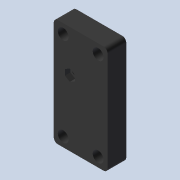
# Autodesk Inventor part: 10_Mountinplate_Mirrors_v1_Combiner
Saved by Autodesk Inventor 2022 (Build 260153000, 153)
## iProperties
Created: 2022-05-18
Part Number: 10_Mountinplate_Mirrors_v1_Combiner
Material: Generisch
Document SubType Name: Modeling
Designer: diederichbenedict
Density: 1 g/cm^3
Appearance: Vorgabe
Author: diederichbenedict
Autodesk Inventor part; units mm, degrees
ref_plane "Arbeitsebene1" through (0.0075, -0.0423, 0) normal (0, 0, 1) x (1, 0, 0)
sketch "Skizze1" plane through (0.0075, -0.0423, 0) normal (0, 0, 1) x (1, 0, 0)
  line L0 (0.635, 25.527) -> (10.16, 25.527) projected
  line L1 (0.635, 25.527) -> (0.635, 0) projected
  line L2 (0.635, 0) -> (10.16, 0) projected
  line L3 (10.16, 0) -> (10.16, 25.527) projected
  line L4 (30.08, -27.3) -> (-3.92, -27.3)
  line L5 (-6.92, -24.3) -> (-6.92, 49.7)
  line L6 (-3.92, 52.7) -> (30.08, 52.7)
  line L7 (33.08, -27.3) -> (-6.92, 52.7) construction
  line L8 (-6.92, -27.3) -> (33.08, 52.7) construction
  arc A0 (30.08, -27.3) -> (33.08, -24.3) centre (30.08, -24.3) ccw
  arc A1 (-6.92, -24.3) -> (-3.92, -27.3) centre (-3.92, -24.3) ccw
  arc A2 (-3.92, 52.7) -> (-6.92, 49.7) centre (-3.92, 49.7) ccw
  arc A3 (33.08, 49.7) -> (30.08, 52.7) centre (30.08, 49.7) ccw
  circle A4 centre (5.08, 12.7) radius 2.3813
  line L9 (33.08, -24.3) -> (33.08, 49.7)
  line L10 (5.08, 12.7) -> (5.08, 21.7)
  line L11 (5.08, 12.7) -> (14.08, 12.7) construction
  circle A5 centre (5.08, 21.7) radius 2.3813
  point P0 (-0.0075, 0.0423)
  point P1 (13.08, 12.7)
  dimension "d1" = 80
  dimension "d2" = 3
  dimension "d7" = 0
  dimension "d8" = 8
  dimension "d41" = 9
  dimension "d42" = 90
  constraints: 16 end point, 8 point on circle, 7 tangent, 6 centre point, 6 point on line, 3 equal radius, 2 horizontal, 2 perpendicular, 2 vertical, 1 midpoint, 1 parallel, 2 other
  measures "d1" distance of L8.start L7.end
  measures "d2" radius of A0
  measures "d7" vertical distance of L10.start point (13.08, 12.7)
  measures "d8" distance of point (13.08, 12.7) L10.start
  measures "d41" distance of L10.start L10.end
  measures "d42" angle of L11 L10
ref_plane "Arbeitsebene2" through (291.5074, -13.3966, 8.6065) normal (0, 0, 1) x (0.898794, -0.4383711, 0)
extrude "Extrusion1" add sketch "Skizze1" along normal blind 12.612 contours L0 L3 L2 L1 | L4 A1 L5 A2 L6 A3 L9 A0 | A4
sketch "Skizze3" plane through (0.0075, -0.0423, 0) normal (0, 0, -1) x (-1, 0, 0)
  arc A0 (-30.08, 52.7) -> (-33.08, 49.7) centre (-30.08, 49.7) ccw projected
  line L0 (-33.08, -24.3) -> (-33.08, 49.7) projected
  arc A1 (-33.08, -24.3) -> (-30.08, -27.3) centre (-30.08, -24.3) ccw projected
  line L1 (3.92, -27.3) -> (-30.08, -27.3) projected
  arc A2 (3.92, -27.3) -> (6.92, -24.3) centre (3.92, -24.3) ccw projected
  line L2 (6.92, 49.7) -> (6.92, -24.3) projected
  arc A3 (6.92, 49.7) -> (3.92, 52.7) centre (3.92, 49.7) ccw projected
  line L3 (-30.08, 52.7) -> (3.92, 52.7) projected
  line L4 (-26.08, 45.7) -> (-0.08, 45.7)
  line L5 (-0.08, 45.7) -> (-0.08, -20.3)
  line L6 (-0.08, -20.3) -> (-26.08, -20.3)
  line L7 (-26.08, -20.3) -> (-26.08, 45.7)
  point P0 (0.0075, 0.0423)
  dimension "d9" = 7
  constraints: 8 end point, 3 other
  measures "d9" distance between parallel lines of L0 L7
hole "Bohrung1" at (26.0875, 45.6577, 0) at (26.0875, -20.3423, 0) at (0.0875, -20.3423, 0) at (0.0875, 45.6577, 0) direction (0, 0, 1) diameter 8 depth 15 tip angle 118
sketch "Skizze4" plane through (-6.9125, -24.3423, 0) normal (-1, 0, 0) x (0, 0, 1)
  circle A0 centre (-6.731, 17.9923) radius 7.366 projected
  circle A1 centre (-6.731, 17.9923) radius 9.366
  circle A2 centre (-6.731, 56.05) radius 7.366
  circle A3 centre (-6.731, 56.05) radius 9.366
  line L0 (-6.731, 17.9923) -> (-6.731, 26.9923)
  line L1 (-6.731, 17.9923) -> (2.269, 17.9923) construction
  circle A4 centre (-6.731, 26.9923) radius 9.366
  point P0 (0, 24.3423)
  dimension "d17" = 2
  dimension "d45" = 9
  dimension "d46" = 90
  constraints: 4 centre point, 4 end point, 1 equal radius, 1 horizontal, 1 perpendicular, 1 vertical, 2 other
  measures "d17" radial gap between concentric circles of A0 A1
  measures "d45" distance of L0.start L0.end
  measures "d46" angle of L1 L0
ref_plane "Arbeitsebene3" through (0, -11.176, -49.276) normal (-1, 0, 0) x (0, 0.0000004, 1)
extrude "Extrusion2" cut sketch "Skizze4" against normal up to surface (6.9125 mm away) contours A4 A0 | A0 A4 A1 | A1 A4 picked at (-6.731, 20.2469) picked at (0.3309, 22.9964)
sketch "Skizze5" plane through (0.0075, -0.0423, 0) normal (0, 0, -1) x (-1, 0, 0)
  line L0 (0.0075, -3.8204) -> (0.0075, 9.2051) projected
  arc A0 (6.92, 49.7) -> (3.92, 52.7) centre (3.92, 49.7) ccw projected
  line L1 (-30.08, 52.7) -> (3.92, 52.7) projected
  arc A1 (-30.08, 52.7) -> (-33.08, 49.7) centre (-30.08, 49.7) ccw projected
  line L2 (-33.08, -24.3) -> (-33.08, 49.7) projected
  arc A2 (-33.08, -24.3) -> (-30.08, -27.3) centre (-30.08, -24.3) ccw projected
  line L3 (3.92, -27.3) -> (-30.08, -27.3) projected
  arc A3 (3.92, -27.3) -> (6.92, -24.3) centre (3.92, -24.3) ccw projected
  line L4 (6.92, 49.7) -> (6.92, 9.2051) projected
  circle A4 centre (-0.08, 45.7) radius 4 projected
  circle A5 centre (-26.08, -20.3) radius 4 projected
  circle A6 centre (-26.08, 45.7) radius 4 projected
  circle A7 centre (-0.08, -20.3) radius 4 projected
  line L5 (-0.6275, 29.1761) -> (-10.1525, 29.1761) projected
  line L6 (-0.6275, -2.2391) -> (-10.1525, -2.2391) projected
  line L7 (-10.1525, -2.2391) -> (-10.1525, 29.1761)
  line L8 (-0.6275, 29.1761) -> (-0.6275, -2.2391)
  line L9 (0.0075, 0.2051) -> (0.0075, -12.8204) projected
  line L10 (-10.3525, 29.3761) -> (-0.4275, 29.3761)
  line L11 (-0.4275, 29.3761) -> (-0.4275, -2.4391)
  line L12 (-0.4275, -2.4391) -> (-10.3525, -2.4391)
  line L13 (-10.3525, -2.4391) -> (-10.3525, 29.3761)
  line L14 (6.92, -3.8204) -> (6.92, -24.3) projected
  line L15 (-12.6873, 36.83) -> (-19.1643, 36.83)
  line L16 (-12.6873, -11.811) -> (-19.1643, -11.811)
  line L17 (-12.6873, 17.399) -> (-12.6873, 4.5974)
  line L18 (-19.7993, 21.1275) -> (-19.7993, 26.543)
  line L19 (-12.6873, -11.811) -> (-19.7993, -11.811)
  line L20 (-19.7993, -11.811) -> (-19.7993, 36.83)
  line L21 (-19.7993, 36.83) -> (-12.6873, 36.83)
  line L22 (-12.6873, 36.83) -> (-12.6873, -11.811)
  line L23 (-19.9993, 37.03) -> (-19.9993, -12.011)
  line L24 (-19.9993, -12.011) -> (-12.4873, -12.011)
  line L25 (-12.4873, -12.011) -> (-12.4873, 37.03)
  line L26 (-12.4873, 37.03) -> (-19.9993, 37.03)
  line L27 (-19.9993, -12.011) -> (-22.9993, -12.011)
  line L28 (-22.9993, -12.011) -> (-22.9993, 37.03)
  line L29 (-22.9993, 37.03) -> (-19.9993, 37.03)
  line L30 (-19.9993, 37.03) -> (-19.9993, -12.011)
  line L31 (0, -0.127) -> (0, 25.4)
  line L32 (0, -0.127) -> (0, 25.4)
  line L33 (-0.4275, -2.4391) -> (0.0075, -2.4391)
  line L34 (0.2725, 0.2051) -> (0.2725, 25.2373)
  line L35 (0.2725, 29.3761) -> (-0.4275, 29.3761)
  line L36 (-0.4275, 29.3761) -> (-0.4275, -2.4391)
  line L37 (0, 6.611) -> (-10.36, 6.611)
  line L38 (-10.36, 6.611) -> (-10.36, 38.411)
  line L39 (-10.36, 38.411) -> (0, 38.411)
  line L40 (0, 38.411) -> (0, 6.611)
  line L41 (6.92, 49.7) -> (6.92, 9.2051) projected
  line L42 (0.0075, 6.98) -> (0.0075, -2.82)
  line L43 (-10.36, 38.411) -> (-12.4873, 38.411)
  line L44 (-12.4873, 39.411) -> (-12.4873, -2.4391)
  line L45 (-10.36, -2.4391) -> (-10.36, 39.411)
  line L46 (-12.4873, 39.411) -> (-12.4873, 7.611)
  line L47 (-12.4873, 6.611) -> (-10.36, 6.611)
  line L48 (-10.36, 7.611) -> (-10.36, 39.411)
  line L49 (-12.4873, 48) -> (-22.9993, 48)
  line L50 (-22.9993, 48) -> (-22.9993, -3)
  line L51 (-22.9993, -3) -> (-12.4873, -3)
  line L52 (-12.4873, -3) -> (-12.4873, 48)
  line L53 (6.92, -3.8204) -> (0.0075, -3.8204) projected
  line L54 (0.0075, 9.2051) -> (6.92, 9.2051) projected
  line L55 (0, 39.411) -> (0, 38.411)
  point P0 (6.92, 0.2051)
  point P1 (6.92, 25.2373)
  point P2 (-19.9993, 37.03)
  point P3 (0, 29.3761)
  point P4 (-10.3525, 6.611)
  point P5 (0, 6.611)
  point P6 (-10.36, 6.611)
  point P7 (-22.9993, -13)
  point P8 (-19.9993, 37.03)
  point P9 (-19.9993, 37.03)
  point P10 (-12.4873, 6.611)
  point P11 (-22.9993, 43.1487)
  point P12 (-22.9993, 48.2513)
  point P13 (-12.4873, -3)
  point P14 (-19.9993, -3)
  point P15 (-12.4873, 6.611)
  point P16 (0, 6.611)
  dimension "d20" = 0.2
  dimension "d26" = 0.2
  dimension "d27" = 3
  dimension "d28" = 0.7
  dimension "d36" = 10.36
  dimension "d37" = 31.8
  dimension "d44" = 51
  dimension "d47" = 1
  constraints: 88 end point, 15 parallel, 8 horizontal, 7 perpendicular, 5 vertical, 4 point on line, 16 other
  measures "d20" distance between parallel lines of L8 L11
  measures "d26" distance between parallel lines of L20 L23
  measures "d27" distance of L28.end L29.end
  measures "d28" distance of L35.end L35.start
  measures "d36" distance of L38.end L39.end
  measures "d37" distance of L37.end L38.end
  measures "d44" distance of L50.end L49.end
  measures "d47" distance of L55.start L55.end
ref_plane "Arbeitsebene4" through (-0.1034, 27.5049, -1.27) normal (0, 0.0000004, 1) x (1, 0, 0)
extrude "Extrusion3" add sketch "Skizze5" along normal up to surface (1.27 mm away) contours L53 L14 A3 L3 A2 L2 A1 L1 A0 L4 L54 L0 | A4 | A5 | L49 L50 A6 | L51 L23 L27 L28 | L51 L20 L19 L16 L22 L25 L24 L23 | L51 L22 L16 L19 L20 | L37 L7 L6 L8 L11 L12 L13 | L37 L8 L6 L7 | A7 picked at (-27.2623, 45.0103)
sketch "Sketch6" plane through (0.0075, -0.0423, 12.612) normal (0, 0, 1) x (1, 0, 0)
  circle A0 centre (5.08, 12.7) radius 2.3813 projected
  line L0 (8.8085, 14.7861) -> (8.7509, 10.5141)
  line L1 (8.7509, 10.5141) -> (5.0224, 8.428)
  line L2 (5.0224, 8.428) -> (1.3515, 10.6139)
  line L3 (1.3515, 10.6139) -> (1.4091, 14.8859)
  line L4 (1.4091, 14.8859) -> (5.1376, 16.972)
  line L5 (5.1376, 16.972) -> (8.8085, 14.7861)
  line L6 (5.08, 12.7) -> (5.08, 21.7)
  line L7 (5.08, 12.7) -> (14.08, 12.7) construction
  line L8 (8.8085, 23.7861) -> (8.7509, 19.5141)
  line L9 (8.7509, 19.5141) -> (5.0224, 17.428)
  line L10 (5.0224, 17.428) -> (1.3515, 19.6139)
  line L11 (1.3515, 19.6139) -> (1.4091, 23.8859)
  line L12 (1.4091, 23.8859) -> (5.1376, 25.972)
  line L13 (5.1376, 25.972) -> (8.8085, 23.7861)
  point P0 (-0.0075, 0.0423)
  point P1 (5.08, 22.7)
  dimension "d23" = 3.7
  dimension "d39" = 9
  dimension "d40" = 90
  constraints: 28 end point, 1 coincident, 1 horizontal, 1 perpendicular, 1 vertical, 14 other
  measures "d23" distance from line of L4 A0.centre
  measures "d39" distance of L6.start L6.end
  measures "d40" angle of L7 L6
extrude "Extrusion4" cut sketch "Sketch6" against normal blind 4 contours L8 L9 L10 L11 L12 L13
sketch "Sketch7" plane through (30.0875, 52.6577, -1.27) normal (0, -0.0000004, -1) x (-1, 0, 0)
  circle A0 centre (30, -73) radius 4 projected
  circle A1 centre (4, -73) radius 4 projected
  circle A2 centre (30, -7) radius 4 projected
  arc A3 (7.0807, -9.5513) -> (7.0807, -4.4487) centre (4, -7) ccw projected
  circle A4 centre (30, -73) radius 6.5
  circle A5 centre (4, -73) radius 6.5
  circle A6 centre (30, -7) radius 6.5
  circle A7 centre (4, -7) radius 6.5
  point P0 (30.0875, -52.6577)
  dimension "d30" = 13
  dimension "d31" = 13
  dimension "d32" = 13
  dimension "d33" = 13
  constraints: 4 centre point, 4 coincident
  measures "d30" diameter of A4
  measures "d31" diameter of A5
  measures "d32" diameter of A6
  measures "d33" diameter of A7
extrude "Extrusion5" cut sketch "Sketch7" against normal blind 8 contours A0 | A1 | A2 | A4 | A5 | A6 | A7
fillet "Fillet1" radius 0.5 7 edges at (23.0068, 18.4459, -1.27) (12.4948, 1.7632, -1.27) (17.7508, -3.0423, -1.27) (6.2511, 6.5687, -1.27) (0.0075, 22.4687, -1.27) (6.2511, 38.3687, -1.27) (16.2514, 47.9577, -1.27)
